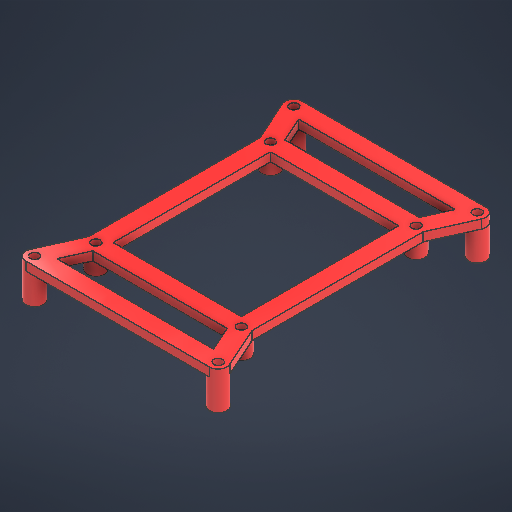
# Autodesk Inventor part: RP_mounting_cover
Saved by Autodesk Inventor 2026.1 (Build 301233000, 233)
## iProperties
Created: 2026-03-24
Part Number: RP_mounting_cover
Material: Generic
Document SubType Name: Modeling
Designer: emanuel
Density: 1 g/cm^3
Appearance: Default
Author: emanuel
Autodesk Inventor part; units mm, degrees
ref_plane "YZ Plane" through (0, 0, 0) normal (1, 0, 0) x (0, 1, 0)
ref_plane "XZ Plane" through (0, 0, 0) normal (0, 1, 0) x (-1, 0, 0)
ref_plane "XY Plane" through (0, 0, 0) normal (0, 0, 1) x (1, 0, 0)
sketch "Sketch1" plane through (0, 0, 0) normal (0, 1, 0) x (-1, 0, 0)
  line L0 (0, 0) -> (63, 0)
  line L1 (63, 0) -> (63, -89)
  line L2 (63, -89) -> (0, -89)
  line L3 (0, -89) -> (0, 0)
  circle A0 centre (0, 0) radius 1.5
  circle A1 centre (63, 0) radius 1.5
  circle A2 centre (0, -89) radius 1.5
  circle A3 centre (63, -89) radius 1.5
  circle A4 centre (0, 0) radius 3
  circle A5 centre (0, -89) radius 3
  circle A6 centre (63, -89) radius 3
  circle A7 centre (63, 0) radius 3
  dimension "d0" = 63
  dimension "d1" = 89
  dimension "d2" = 3
  dimension "d3" = 3
  dimension "d4" = 3
  dimension "d5" = 3
  dimension "d6" = 6
  dimension "d7" = 6
  dimension "d8" = 6
  dimension "d9" = 6
  constraints: 8 centre point, 8 coincident, 8 end point, 2 parallel, 1 horizontal, 1 perpendicular
  measures "d0" distance of L1.end L2.end
  measures "d1" distance of L0.end L1.end
  measures "d2" diameter of A0
  measures "d3" diameter of A1
  measures "d4" diameter of A2
  measures "d5" diameter of A3
  measures "d6" diameter of A4
  measures "d7" diameter of A5
  measures "d8" diameter of A6
  measures "d9" diameter of A7
extrude "Extrusion1" add sketch "Sketch1" along normal blind 10 contours A0 L3 A4 L0 | L0 A4 L3 A0 | A7 L1 A1 L0 | L0 A1 L1 A7 | A5 L2 A2 L3 | L3 A2 L2 A5 | A6 L2 A3 L1 | L1 A3 L2 A6
sketch "Sketch2" plane through (0, 10, 0) normal (0, 1, 0) x (1, 0, 0)
  circle A0 centre (0, 0) radius 1.5 projected
  circle A1 centre (-63, 89) radius 1.5 projected
  line L0 (0, 0) -> (-63, 0)
  line L1 (-63, 0) -> (-63, 89)
  line L2 (-63, 89) -> (0, 89)
  line L3 (0, 89) -> (0, 0)
  line L4 (-63, 44.5) -> (-31.5, 44.5)
  line L5 (-6.5, 14.5) -> (-56.5, 14.5)
  line L6 (-56.5, 14.5) -> (-56.5, 74.5)
  line L7 (-56.5, 74.5) -> (-6.5, 74.5)
  line L8 (-6.5, 74.5) -> (-6.5, 14.5)
  line L9 (-6.5, 14.5) -> (-56.5, 74.5) construction
  line L10 (-56.5, 14.5) -> (-6.5, 74.5) construction
  circle A2 centre (-56.5, 14.5) radius 1.5
  circle A3 centre (-6.5, 14.5) radius 1.5
  circle A4 centre (-6.5, 74.5) radius 1.5
  circle A5 centre (-56.5, 74.5) radius 1.5
  circle A6 centre (-56.5, 14.5) radius 3
  circle A7 centre (-56.5, 74.5) radius 3
  circle A8 centre (-6.5, 14.5) radius 3
  circle A9 centre (-6.5, 74.5) radius 3
  dimension "d12" = 50
  dimension "d13" = 60
  dimension "d14" = 3
  dimension "d15" = 3
  dimension "d16" = 3
  dimension "d17" = 3
  dimension "d18" = 6
  dimension "d19" = 6
  dimension "d20" = 6
  dimension "d21" = 6
  constraints: 22 end point, 8 centre point, 8 coincident, 4 parallel, 3 horizontal, 3 midpoint, 2 perpendicular
  measures "d12" distance of L6.end L7.end
  measures "d13" distance of L5.end L6.end
  measures "d14" diameter of A2
  measures "d15" diameter of A3
  measures "d16" diameter of A4
  measures "d17" diameter of A5
  measures "d18" diameter of A6
  measures "d19" diameter of A7
  measures "d20" diameter of A8
  measures "d21" diameter of A9
extrude "Extrusion2" add sketch "Sketch2" against normal blind 5 contours A6 L6 A2 L5 | L5 A2 L6 A6 | A8 L8 A3 L5 | L5 A3 L8 A8 | A9 L7 A4 L8 | L8 A4 L7 A9 | A7 L7 A5 L6 | L6 A5 L7 A7
sketch "Sketch3" plane through (-63, 10, 0) normal (0, 1, 0) x (1, 0, 0)
  circle A0 centre (0, 0) radius 1.5 projected
  circle A1 centre (6.5, 14.5) radius 1.5 projected
  line L0 (0, 0) -> (6.5, 14.5) construction
  line L1 (2.7375, -1.2272) -> (9.2375, 13.2728)
  line L2 (3.7625, 15.7272) -> (-2.7375, 1.2272)
  arc A2 (-2.7375, 1.2272) -> (2.7375, -1.2272) centre (0, 0) ccw
  arc A3 (9.2375, 13.2728) -> (3.7625, 15.7272) centre (6.5, 14.5) ccw
  circle A4 centre (6.5, 74.5) radius 1.5 projected
  line L3 (6.5, 14.5) -> (6.5, 74.5) construction
  line L4 (3.5, 14.5) -> (3.5, 74.5)
  line L5 (9.5, 74.5) -> (9.5, 14.5)
  arc A5 (3.5, 14.5) -> (9.5, 14.5) centre (6.5, 14.5) ccw
  arc A6 (9.5, 74.5) -> (3.5, 74.5) centre (6.5, 74.5) ccw
  circle A7 centre (0, 89) radius 1.5 projected
  line L6 (6.5, 74.5) -> (0, 89) construction
  line L7 (3.7705, 73.2764) -> (-2.7295, 87.7764)
  line L8 (2.7295, 90.2236) -> (9.2295, 75.7236)
  arc A8 (3.7705, 73.2764) -> (9.2295, 75.7236) centre (6.5, 74.5) ccw
  arc A9 (2.7295, 90.2236) -> (-2.7295, 87.7764) centre (0, 89) ccw
  circle A10 centre (63, 89) radius 1.5 projected
  line L9 (0, 89) -> (63, 89) construction
  line L10 (0, 86.0176) -> (63, 86.0176)
  line L11 (63, 91.9824) -> (0, 91.9824)
  arc A11 (0, 91.9824) -> (0, 86.0176) centre (0, 89) ccw
  arc A12 (63, 86.0176) -> (63, 91.9824) centre (63, 89) ccw
  circle A13 centre (56.5, 74.5) radius 1.5 projected
  line L12 (63, 89) -> (56.5, 74.5) construction
  line L13 (60.2705, 90.2236) -> (53.7705, 75.7236)
  line L14 (59.2295, 73.2764) -> (65.7295, 87.7764)
  arc A14 (65.7295, 87.7764) -> (60.2705, 90.2236) centre (63, 89) ccw
  arc A15 (53.7705, 75.7236) -> (59.2295, 73.2764) centre (56.5, 74.5) ccw
  circle A16 centre (56.5, 14.5) radius 1.5 projected
  line L15 (56.5, 74.5) -> (56.5, 14.5) construction
  line L16 (53.5, 74.5) -> (53.5, 14.5)
  line L17 (59.5, 14.5) -> (59.5, 74.5)
  arc A17 (59.5, 74.5) -> (53.5, 74.5) centre (56.5, 74.5) ccw
  arc A18 (53.5, 14.5) -> (59.5, 14.5) centre (56.5, 14.5) ccw
  line L18 (56.5, 14.5) -> (63, 0) construction
  line L19 (53.7705, 13.2764) -> (60.2705, -1.2236)
  line L20 (65.7295, 1.2236) -> (59.2295, 15.7236)
  arc A19 (59.2295, 15.7236) -> (53.7705, 13.2764) centre (56.5, 14.5) ccw
  arc A20 (60.2705, -1.2236) -> (65.7295, 1.2236) centre (63, 0) ccw
  line L21 (63, 0) -> (0, 0) construction
  line L22 (63, 3) -> (0, 3)
  line L23 (0, -3) -> (63, -3)
  arc A21 (63, -3) -> (63, 3) centre (63, 0) ccw
  arc A22 (0, 3) -> (0, -3) centre (0, 0) ccw
  line L24 (6.5, 14.5) -> (56.5, 14.5) construction
  line L25 (6.5, 11.5176) -> (56.5, 11.5176)
  line L26 (56.5, 17.4824) -> (6.5, 17.4824)
  arc A23 (6.5, 17.4824) -> (6.5, 11.5176) centre (6.5, 14.5) ccw
  arc A24 (56.5, 11.5176) -> (56.5, 17.4824) centre (56.5, 14.5) ccw
  line L27 (6.5, 74.5) -> (56.5, 74.5) construction
  line L28 (6.5, 77.5) -> (56.5, 77.5)
  line L29 (56.5, 71.5) -> (6.5, 71.5)
  arc A25 (6.5, 77.5) -> (6.5, 71.5) centre (6.5, 74.5) ccw
  arc A26 (56.5, 71.5) -> (56.5, 77.5) centre (56.5, 74.5) ccw
  circle A27 centre (63, 0) radius 1.5 projected
  circle A28 centre (63, 0) radius 1.5
  circle A29 centre (63, 89) radius 1.5
  circle A30 centre (0, 89) radius 1.5
  point P0 (3.25, 7.25)
  point P1 (6.5, 44.5)
  point P2 (3.25, 81.75)
  point P3 (31.5, 89)
  point P4 (59.75, 81.75)
  point P5 (56.5, 44.5)
  point P6 (59.75, 7.25)
  point P7 (31.5, 0)
  point P8 (31.5, 14.5)
  point P9 (31.5, 74.5)
  point P10 (0.2294, 91.9824)
  point P11 (3.5, 73.8799)
  point P12 (3.5, 15.1417)
  point P13 (65.6357, 1.4329)
  point P14 (59.5, 15.1202)
  point P15 (59.5, 73.8799)
  point P16 (62.7706, 91.9824)
  point P17 (54.5589, 11.5176)
  point P18 (58.3772, 3)
  point P19 (4.6325, 3)
  point P20 (8.4507, 11.5176)
  point P21 (53.5, 17.4824)
  point P22 (9.5, 17.4824)
  point P23 (9.5, 71.5)
  point P24 (53.5, 71.5)
  point P25 (4.6149, 86.0176)
  point P26 (58.3851, 86.0176)
  point P27 (54.5669, 77.5)
  point P28 (8.4331, 77.5)
  point P29 (3.5, 22.3126)
  point P30 (9.5, 14.5)
  point P31 (9.1353, 75.9335)
  point P32 (53.8647, 75.9335)
  point P33 (53.8643, 13.0671)
  point P34 (7.8263, -3)
  point P35 (14.3193, 11.5176)
  point P36 (6.8244, 17.4824)
  point P37 (56.2706, 17.4824)
  point P38 (3.6764, 73.4864)
  point P39 (6.2021, 82.4768)
  point P40 (56.7979, 82.4768)
  point P41 (59.3236, 73.4864)
  dimension "d26" = 6
  dimension "d27" = 6
  constraints: 80 end point, 40 point on circle, 40 tangent, 23 centre point, 12 parallel, 10 midpoint, 5 perpendicular, 3 coincident, 2 concentric, 1 vertical
  measures "d26" distance between parallel lines of L2 L1
  measures "d27" distance between parallel lines of L29 L28
extrude "Extrusion3" add sketch "Sketch3" along normal blind 3 contours A2 A22 L22 L1 | L1 L22 L19 A20 L20 A21 L23 A2 | L22 A22 L2 L4 A5 L25 L1 | L25 A5 L1 | L1 A3 L5 L26 L16 A18 L19 L25 | L22 A21 L20 A20 L19 | L19 L25 A18 L17 L20 A21 L22 | A5 L25 A23 L26 A3 | A5 L4 L2 A3 L26 A23 L25 | L19 A18 L25 | L4 L7 A25 L29 L5 L26 A3 L2 | A3 L26 L5 | L19 A19 L26 A24 L25 A18 | A18 L16 L26 A19 L19 | L25 A24 L26 A19 L20 L17 A18 | L7 A9 L11 A11 L10 L8 L28 A6 L4 | L4 A25 L7 | L20 A19 L26 L16 L29 A26 L14 L17 | A6 L8 A8 L7 A25 | L7 A8 L8 A6 L5 L29 A25 | L17 A17 L28 L13 L10 A12 L11 A14 L14 | L14 A26 L17 | L5 A6 L8 L28 L13 A17 L16 L29 | L28 L8 A6 | L11 A14 L13 L10 L8 A9 | A9 L8 L10 A11 L11 | A26 L29 L16 A17 L13 A15 L14 | L14 A15 L13 A17 A26 | L11 A12 L10 L13 A14 | A17 L13 L28
body "Solid1"
